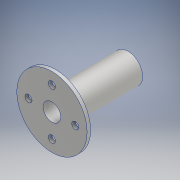
# Autodesk Inventor part: Hub_v4
Saved by Autodesk Inventor 2018 (Build 220112000, 112)
## iProperties
Created: 2017-10-24
Part Number: Hub_v4
Material: アルミニウム 6061
Document SubType Name: Modeling
Designer: 翔
Density: 2.7 g/cm^3
Appearance: アルミニウム - フラット
Author: 翔
Autodesk Inventor part; units mm, degrees
ref_plane "YZ Plane" through (0, 0, 0) normal (1, 0, 0) x (0, 1, 0)
ref_plane "XZ Plane" through (0, 0, 0) normal (0, 1, 0) x (-1, 0, 0)
ref_plane "XY Plane" through (0, 0, 0) normal (0, 0, 1) x (1, 0, 0)
sketch "スケッチ1" plane through (0, 0, 0) normal (0, 0, 1) x (1, 0, 0)
  line L0 (-6, 0) -> (36, 0) projected
  line L1 (0, -13) -> (0, 78) projected
  line L2 (7.5, 0) -> (30, 0)
  line L3 (30, 3) -> (12.5, 3)
  line L4 (12.5, 3) -> (12.5, 65)
  line L5 (12.5, 65) -> (7.5, 65)
  line L6 (7.5, 65) -> (7.5, 0)
  line L7 (30, 3) -> (30, 0)
  point P0 (0, 0)
  dimension "d0" = 7.5
  dimension "d1" = 5
  dimension "d2" = 30
  dimension "d3" = 65
  dimension "d4" = 3
  constraints: 12 end point, 4 perpendicular, 1 horizontal
  measures "d0" distance between parallel lines of L6 L1
  measures "d1" distance between parallel lines of L6 L4
  measures "d2" distance between parallel lines of L1 L7
  measures "d3" distance between parallel lines of L5 L0
  measures "d4" distance between parallel lines of L2 L3
revolve "回転1" add sketch "スケッチ1" angle 360 about axis through (0, -10, 0) along (0, 1, 0)
sketch "スケッチ2" plane through (0, 0, 0) normal (0, -1, 0) x (1, 0, 0)
  circle A0 centre (0, 0) radius 20
  line L0 (-42, 0) -> (42, 0) projected
  line L1 (0, -42) -> (0, 42) projected
  circle A1 centre (20, 0) radius 3
  circle A2 centre (0, 20) radius 3
  circle A3 centre (-20, 0) radius 3
  circle A4 centre (0, -20) radius 3
  dimension "d6" = 40
  dimension "d7" = 6
  dimension "d10" = 360
  constraints: 4 centre point, 1 coincident, 1 horizontal alignment, 1 point on line, 11 other
  measures "d7" diameter of A1
extrude "押し出し1" cut sketch "スケッチ2" against normal blind 10 contours L0 A1 A0 | L0 A1 A0 | A0 A1 L0 | A0 A1 L0 | A2 L1 A0 | A0 L1 A2 | A4 L1 A0 | A0 L1 A4 | L1 A2 A0 | A0 A2 L1 | L1 A4 A0 | A0 A4 L1 | A3 A0 L0 | L0 A0 A3 | L0 A3 A0 | A0 A3 L0
sketch "スケッチ3" plane through (0, 65, 0) normal (0, 1, 0) x (1, 0, 0)
  line L0 (0, 42) -> (0, -42) projected
  line L1 (-42, 0) -> (42, 0) projected
  circle A0 centre (0, 0) radius 7.5 projected
  line L2 (2.5, -9.5011) -> (-2.5, -9.5011)
  line L3 (-2.5, -9.5011) -> (-2.5, -7.0711)
  line L4 (2.5, -7.0711) -> (2.5, -9.5011)
  line L5 (2.5, -9.5011) -> (-2.5, -7.0711) construction
  line L6 (-2.5, -9.5011) -> (2.5, -7.0711) construction
  circle A1 centre (0, 0) radius 12.5 projected
  circle A2 centre (0, 0) radius 7.5 projected
  circle A3 centre (0, 0) radius 7.5 projected
  arc A4 (-2.5, -7.0711) -> (2.5, -7.0711) centre (0, 0) ccw
  point P0 (0, -8.2861)
  dimension "d15" = 5
  dimension "d17" = 2.43
  constraints: 10 end point, 2 midpoint, 2 point on circle, 1 centre point, 1 coincident, 1 concentric, 1 horizontal, 1 parallel, 1 perpendicular, 1 point on line, 2 other
  measures "d15" distance of L2.start L2.end
  measures "d17" distance of L4.start L2.start
extrude "押し出し2" cut sketch "スケッチ3" against normal blind 20 contours A0 L4 L2 L0 | L0 L2 L3 A0
